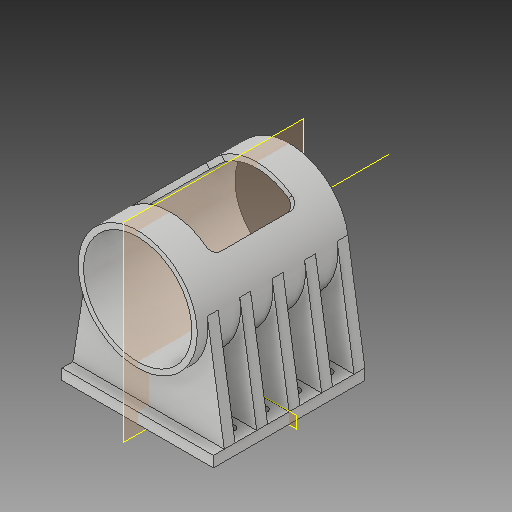
# Autodesk Inventor part: LENS MOUNT
Saved by Autodesk Inventor 2017 (Build 210142000, 142)
## iProperties
Created: 2017-04-01
Part Number: LENS MOUNT
Material: Generic
Document SubType Name: Modeling
Designer: Muchen
Density: 1 g/cm^3
Appearance: Default
Mass: 89.8055 g
Surface Area: 473.168 cm^2
Volume: 89.8055 cm^3
Author: Muchen
Autodesk Inventor part; units mm, degrees
ref_plane "YZ Plane" through (0, 0, 0) normal (1, 0, 0) x (0, 1, 0)
ref_plane "XZ Plane" through (0, 0, 0) normal (0, 1, 0) x (-1, 0, 0)
ref_plane "XY Plane" through (0, 0, 0) normal (0, 0, 1) x (1, 0, 0)
sketch "Sketch1" plane through (0, 0, 0) normal (0, 1, 0) x (-1, 0, 0)
  line L0 (0, 0) -> (70, 0)
  line L1 (70, 0) -> (70, -70)
  line L2 (70, -70) -> (0, -70)
  line L3 (0, -70) -> (0, 0)
  dimension "d0" = 70
  dimension "d1" = 70
  constraints: 8 end point, 2 parallel, 1 horizontal, 1 perpendicular
  measures "d0" distance of L1.end L2.end
  measures "d1" distance of L2.end L0.start
extrude "Extrusion1" add sketch "Sketch1" along normal blind 5
ref_plane "Work Plane2" through (-70, 0, -35) normal (0, 0, 1) x (1, 0, 0)
sketch "Sketch2" plane through (-70, 0, -35) normal (0, 0, 1) x (1, 0, 0)
  circle A0 centre (35, 50) radius 25
  line L0 (35, 50) -> (35, 5) construction
  line L1 (70, 5) -> (0, 5)
  circle A1 centre (35, 50) radius 27.5
  line L2 (0, 5) -> (7.8411, 54.318)
  line L3 (70, 5) -> (62.1589, 54.318)
  line L4 (0, 0) -> (70, 0) projected
  dimension "d4" = 50
  dimension "d6" = 55
  dimension "d22" = 50
  constraints: 8 end point, 4 coincident, 2 centre point, 2 point on circle, 2 tangent, 1 midpoint, 1 vertical
  measures "d4" diameter of A0
  measures "d6" diameter of A1
  measures "d22" distance from line of L4 L0.start
extrude "Extrusion2" add sketch "Sketch2" against normal blind 5 contours L1 L2 A1 L3
pattern_linear "Rectangular Pattern1" count 5 spacing 15 along (0, 0, -1) of "Extrusion2" first direction both ways yes
extrude "Extrusion3" add sketch "Sketch2" along normal mid plane 70 contours A1
ref_plane "Work Plane1" through (-35, 0, 0) normal (1, 0, 0) x (0, 0, -1)
sketch "Sketch3" plane through (-35, 0, 0) normal (1, 0, 0) x (0, 0, -1)
  line L0 (70, 75) -> (0, 75) projected
  line L1 (70, 77.5) -> (0, 77.5) projected
  line L2 (15, 75) -> (55, 75)
  line L3 (55, 75) -> (55, 77.5)
  line L4 (55, 77.5) -> (15, 77.5)
  line L5 (15, 77.5) -> (15, 75)
  line L6 (84, 50) -> (-14, 50) projected
  point P0 (0, 0)
  dimension "d19" = 15
  dimension "d20" = 15
  constraints: 8 end point, 2 parallel, 2 point on line, 1 horizontal, 1 perpendicular
  measures "d19" distance from line of L1.start L3
  measures "d20" distance from line of L1.end L5
revolve "Revolution1" cut sketch "Sketch3" angle 90 mid plane about axis through (-35, 50, -35) along (0, 0, 1)
fillet "Fillet1" radius 4 4 edges at (-16.4384, 68.5616, -55) (-53.5616, 68.5616, -55) (-53.5616, 68.5616, -15) (-16.4384, 68.5616, -15)
sketch "Sketch4" plane through (0, 0, 0) normal (0, -1, 0) x (1, 0, 0)
  line L0 (0, -65) -> (-70, -65) projected
  line L1 (-70, -65) -> (-70, -55) projected
  line L2 (-70, -55) -> (0, -55) projected
  line L3 (0, -55) -> (0, -65) projected
  line L4 (0, -50) -> (-70, -50) projected
  line L5 (-70, -50) -> (-70, -40) projected
  line L6 (-70, -40) -> (0, -40) projected
  line L7 (0, -40) -> (0, -50) projected
  line L8 (-70, -25) -> (0, -25) projected
  line L9 (0, -25) -> (0, -35) projected
  line L10 (0, -35) -> (-70, -35) projected
  line L11 (-70, -35) -> (-70, -25) projected
  line L12 (0, -20) -> (-70, -20) projected
  line L13 (-70, -20) -> (-70, -10) projected
  line L14 (-70, -10) -> (0, -10) projected
  line L15 (0, -10) -> (0, -20) projected
  line L16 (0, 0) -> (-70, 0) construction
  line L17 (-7, 0) -> (-7, -70) construction
  line L18 (-70, -70) -> (0, -70) construction
  line L19 (-70, 0) -> (0, 0) construction
  line L20 (-63, 0) -> (-63, -70) construction
  line L21 (0, -70) -> (0, 0) construction
  line L22 (-70, 0) -> (-70, -70) construction
  point P0 (-7, -60)
  point P1 (0, -60)
  dimension "d23" = 7
  dimension "d24" = 7
  constraints: 4 end point, 4 point on line, 2 vertical, 1 horizontal alignment, 1 midpoint, 2 other
  measures "d23" distance of the line from the sketch origin of L17
hole "Hole1" at (-7, 0, -60) direction (0, 1, 0) diameter 4 depth 9.525
pattern_linear "Rectangular Pattern2" count 4 spacing 15 along (0, 0, 1) of "Hole1"
mirror "Mirror1" about plane through (-35, 0, 0) normal (1, 0, 0) of "Hole1", "Rectangular Pattern2"
body "Solid1"
